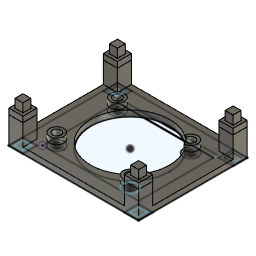
joyhv2 (Autodesk Fusion 360 design; units mm, degrees)
Autodesk Fusion 360 part; units mm, degrees
sketch "Sketch1" plane through (0, 0, 0) normal (0, 0, 1) x (1, 0, 0)
  line L0 (0, 0) -> (34, 0)
  line L1 (34, 0) -> (34, 26.5)
  line L2 (34, 26.5) -> (0, 26.5)
  line L3 (0, 26.5) -> (0, 0)
  line L4 (0, 26.5) -> (34, 26.5)
  line L5 (34, 26.5) -> (34, 28)
  line L6 (34, 28) -> (0, 28)
  line L7 (0, 28) -> (0, 26.5)
  circle A0 centre (28.5, 24) radius 1.5
  circle A1 centre (28.5, 2.5) radius 1.5
  circle A2 centre (2.5, 2.5) radius 1.5
  circle A3 centre (2.5, 24) radius 1.5
  circle A4 centre (16.5, 14.5) radius 14
  line L8 (-6, 32.5) -> (40, 32.5)
  line L9 (40, 32.5) -> (40, -6)
  line L10 (40, -6) -> (-6, -6)
  line L11 (-6, -6) -> (-6, 32.5)
  line L12 (40, 32.5) -> (35, 32.5)
  line L13 (35, 32.5) -> (35, 27.5)
  line L14 (35, 27.5) -> (40, 27.5)
  line L15 (40, 27.5) -> (40, 32.5)
  line L16 (40, -6) -> (35, -6)
  line L17 (35, -6) -> (35, -1)
  line L18 (35, -1) -> (40, -1)
  line L19 (40, -1) -> (40, -6)
  line L20 (-6, -6) -> (-1, -6)
  line L21 (-1, -6) -> (-1, -1)
  line L22 (-1, -1) -> (-6, -1)
  line L23 (-6, -1) -> (-6, -6)
  line L24 (-6, 32.5) -> (-1, 32.5)
  line L25 (-1, 32.5) -> (-1, 27.5)
  line L26 (-1, 27.5) -> (-6, 27.5)
  line L27 (-6, 27.5) -> (-6, 32.5)
  line L28 (-5, 31.5) -> (-2, 31.5)
  line L29 (-2, 31.5) -> (-2, 28.5)
  line L30 (-2, 28.5) -> (-5, 28.5)
  line L31 (-5, 28.5) -> (-5, 31.5)
  line L32 (-5, -2) -> (-2, -2)
  line L33 (-2, -2) -> (-2, -5)
  line L34 (-2, -5) -> (-5, -5)
  line L35 (-5, -5) -> (-5, -2)
  line L36 (36, -2) -> (39, -2)
  line L37 (39, -2) -> (39, -5)
  line L38 (39, -5) -> (36, -5)
  line L39 (36, -5) -> (36, -2)
  line L40 (36, 31.5) -> (39, 31.5)
  line L41 (39, 31.5) -> (39, 28.5)
  line L42 (39, 28.5) -> (36, 28.5)
  line L43 (36, 28.5) -> (36, 31.5)
  circle A5 centre (28.5, 2.5) radius 2.5
  circle A6 centre (28.5, 24) radius 2.5
  circle A7 centre (2.5, 2.5) radius 2.5
  circle A8 centre (2.5, 24) radius 2.5
  dimension "d1" = 34
  dimension "d2" = 26.5
  dimension "d3" = 1.5
  dimension "d4" = 3
  dimension "d5" = 3
  dimension "d6" = 3
  dimension "d7" = 3
  dimension "d8" = 2.5
  dimension "d9" = 2.5
  dimension "d10" = 2.5
  dimension "d11" = 5.5
  dimension "d12" = 5.5
  dimension "d13" = 2.5
  dimension "d14" = 2.5
  dimension "d15" = 2.5
  dimension "d16" = 28
  dimension "d17" = 16.5
  dimension "d18" = 6
  dimension "d19" = 6
  dimension "d20" = 6
  dimension "d21" = 6
  dimension "d22" = 5
  dimension "d23" = 5
  dimension "d24" = 5
  dimension "d25" = 5
  dimension "d26" = 5
  dimension "d27" = 5
  dimension "d28" = 5
  dimension "d29" = 5
  dimension "d30" = 1
  dimension "d31" = 1
  dimension "d32" = 3
  dimension "d33" = 1
  dimension "d34" = 1
  dimension "d35" = 5
  dimension "d36" = 5
  dimension "d37" = 5
  dimension "d77" = 14.5
  constraint horizontal L0
  constraint vertical L1
  constraint horizontal L2
  constraint vertical L3
  constraint coincident L0.start L3.end
  constraint horizontal L4
  constraint vertical L5
  constraint horizontal L6
  constraint vertical L7
  constraint horizontal L8
  constraint vertical L9
  constraint horizontal L10
  constraint vertical L11
  constraint horizontal L12
  constraint vertical L13
  constraint horizontal L14
  constraint vertical L15
  constraint horizontal L16
  constraint vertical L17
  constraint horizontal L18
  constraint vertical L19
  constraint horizontal L20
  constraint vertical L21
  constraint horizontal L22
  constraint vertical L23
  constraint horizontal L24
  constraint vertical L25
  constraint horizontal L26
  constraint vertical L27
  constraint horizontal L28
  constraint vertical L29
  constraint horizontal L30
  constraint vertical L31
  constraint horizontal L32
  constraint vertical L33
  constraint horizontal L34
  constraint vertical L35
  constraint horizontal L36
  constraint vertical L37
  constraint horizontal L38
  constraint vertical L39
  constraint horizontal L40
  constraint vertical L41
  constraint horizontal L42
  constraint vertical L43
  constraint concentric A1 A5
  constraint concentric A0 A6
  constraint concentric A2 A7
  constraint concentric A3 A8
  measures "d1" distance of L0.start L0.end
  measures "d2" distance of L0.start L2.end
  measures "d3" distance of L2.end L6.end
  measures "d4" diameter of A0
  measures "d5" diameter of A1
  measures "d6" diameter of A2
  measures "d7" diameter of A3
  measures "d8" distance of L2 A3.centre
  measures "d9" distance of L3 A3.centre
  measures "d10" distance of L2 A0.centre
  measures "d11" distance of L1 A0.centre
  measures "d12" distance of L1 A1.centre
  measures "d13" distance of L0 A1.centre
  measures "d14" distance of L0 A2.centre
  measures "d15" distance of L3 A2.centre
  measures "d16" diameter of A4
  measures "d17" distance of L3 A4.centre
  measures "d18" distance of L4 L8
  measures "d19" distance of L3 L11
  measures "d20" distance of L0 L10
  measures "d21" distance of L1 L9
  measures "d22" distance of L8.end L12.end
  measures "d23" distance of L8.end L14.end
  measures "d24" distance of L9.end L16.end
  measures "d25" distance of L9.end L18.end
  measures "d26" distance of L10.end L20.end
  measures "d27" distance of L10.end L22.end
  measures "d28" distance of L8.start L24.end
  measures "d29" distance of L8.start L26.end
  measures "d30" distance of L8 L28
  measures "d31" distance of L27 L31
  measures "d32" distance of L40.start L42.end
  measures "d33" distance of L8 L40
  measures "d34" distance of L13 L43
  measures "d35" diameter of A6
  measures "d36" diameter of A7
  measures "d37" diameter of A8
  measures "d77" distance of L0 A4.centre
extrude "Extrude1" add sketch "Sketch1" along normal blind 2 contours L0 L3 A7 | A5 | L0 L1 L2 L3 L4 A4 A6 A7 A8 | A7 | L2 L3 L4 A8 | A8 | L2 L4 L6 L7 A4 | L2 L4 L5 L6 A4 | L2 L4 A4 A6 | A0 A4 A6 | L8 L11 L24 L25 L26 L27 | L8 L9 L10 L11 L13 L14 L17 L18 L21 L22 L25 L26 | L8 L9 L12 L13 L14 L15 | L10 L11 L20 L21 L22 L23 | L9 L10 L16 L17 L18 L19 | L28 L29 L30 L31 | L32 L33 L34 L35 | L36 L37 L38 L39 | L40 L41 L42 L43 picked at (25.5001, 25.6456) picked at (26.5851, 24.6642) makes body 1
extrude "Extrude2" add sketch "Sketch1" along normal blind 4 contours A5 | A7 | A8 | A0 A4 A6 picked at (26.5851, 24.6642) bodies 1
extrude "Extrude3" add sketch "Sketch1" along normal blind 4 contours L8 L11 L24 L25 L26 L27 | L8 L9 L12 L13 L14 L15 | L10 L11 L20 L21 L22 L23 | L9 L10 L16 L17 L18 L19 | L28 L29 L30 L31 | L32 L33 L34 L35 | L36 L37 L38 L39 | L40 L41 L42 L43 bodies 1
extrude "Extrude4" add sketch "Sketch1" along normal blind 11.5 contours L8 L11 L24 L25 L26 L27 | L8 L9 L12 L13 L14 L15 | L10 L11 L20 L21 L22 L23 | L9 L10 L16 L17 L18 L19 bodies 1
move_body "Move1" bodies 1 to x (1, 0, 0) y (0, 1, 0) z (0, 0, 1) at (-61, 0, 0)
extrude "Extrude5" add sketch "Sketch1" along normal blind 2 separate body contours L0 L3 A7 | A5 | L0 L1 L2 L3 L4 A4 A6 A7 A8 | A7 | L2 L3 L4 A8 | A8 | L2 L4 L6 L7 A4 | L2 L4 L5 L6 A4 | L2 L4 A4 A6 | A0 A4 A6 | A0 A4 | A1 | A2 | A3 | L8 L11 L24 L25 L26 L27 | L8 L9 L10 L11 L13 L14 L17 L18 L21 L22 L25 L26 | L8 L9 L12 L13 L14 L15 | L10 L11 L20 L21 L22 L23 | L9 L10 L16 L17 L18 L19 | L28 L29 L30 L31 | L32 L33 L34 L35 | L36 L37 L38 L39 | L40 L41 L42 L43 picked at (25.5001, 25.6456) picked at (26.5851, 24.6642) picked at (28.192, 23.7895) makes body 2
extrude "Extrude6" add sketch "Sketch1" along normal blind 9.5 contours L8 L11 L24 L25 L26 L27 | L8 L9 L12 L13 L14 L15 | L10 L11 L20 L21 L22 L23 | L9 L10 L16 L17 L18 L19 | L28 L29 L30 L31 | L32 L33 L34 L35 | L36 L37 L38 L39 | L40 L41 L42 L43 bodies 2
sketch "Sketch2" plane through (0, 0, 9.5) normal (0, 0, 1) x (-1, 0, 0)
  line L0 (6, -27.5) -> (1, -27.5)
  line L1 (1, -27.5) -> (1, -32.5)
  line L2 (1, -32.5) -> (6, -32.5)
  line L3 (6, -32.5) -> (6, -27.5)
  line L4 (4.9, -31.4) -> (2.1, -31.4)
  line L5 (2.1, -31.4) -> (2.1, -28.6)
  line L6 (2.1, -28.6) -> (4.9, -28.6)
  line L7 (4.9, -28.6) -> (4.9, -31.4)
  line L8 (6, -27.5) -> (6, -32.5)
  line L9 (6, -32.5) -> (-40, -32.5)
  dimension "d50" = 2.8
  dimension "d51" = 2.8
  dimension "d52" = 1.1
  dimension "d53" = 1.1
  constraint horizontal L4
  constraint vertical L5
  constraint horizontal L6
  constraint vertical L7
  measures "d50" distance of L4.start L4.end
  measures "d51" distance of L4.start L6.end
  measures "d52" distance of L7 L8
  measures "d53" distance of L4 L9
sketch "Sketch3" plane through (0, 0, 9.5) normal (0, 0, 1) x (-1, 0, 0)
  line L0 (-40, -27.5) -> (-40, -32.5)
  line L1 (-40, -32.5) -> (-35, -32.5)
  line L2 (-35, -32.5) -> (-35, -27.5)
  line L3 (-35, -27.5) -> (-40, -27.5)
  line L4 (-36.1, -31.4) -> (-38.9, -31.4)
  line L5 (-38.9, -31.4) -> (-38.9, -28.6)
  line L6 (-38.9, -28.6) -> (-36.1, -28.6)
  line L7 (-36.1, -28.6) -> (-36.1, -31.4)
  line L8 (6, -32.5) -> (-40, -32.5)
  line L9 (-40, -27.5) -> (-40, -32.5)
  dimension "d54" = 2.8
  dimension "d55" = 2.8
  dimension "d56" = 1.1
  dimension "d57" = 1.1
  constraint horizontal L4
  constraint vertical L5
  constraint horizontal L6
  constraint vertical L7
  measures "d54" distance of L4.start L4.end
  measures "d55" distance of L4.start L6.end
  measures "d56" distance of L4 L8
  measures "d57" distance of L5 L9
sketch "Sketch4" plane through (0, 0, 9.5) normal (0, 0, 1) x (-1, 0, 0)
  line L0 (-40, 1) -> (-35, 1)
  line L1 (-35, 1) -> (-35, 6)
  line L2 (-35, 6) -> (-40, 6)
  line L3 (-40, 6) -> (-40, 1)
  line L4 (-36.1, 2.1) -> (-38.9, 2.1)
  line L5 (-38.9, 2.1) -> (-38.9, 4.9)
  line L6 (-38.9, 4.9) -> (-36.1, 4.9)
  line L7 (-36.1, 4.9) -> (-36.1, 2.1)
  line L8 (-35, 1) -> (-40, 1)
  line L9 (-40, -32.5) -> (-40, 6)
  dimension "d58" = 2.8
  dimension "d59" = 2.8
  dimension "d60" = 1.1
  dimension "d61" = 1.1
  constraint horizontal L4
  constraint vertical L5
  constraint horizontal L6
  constraint vertical L7
  measures "d58" distance of L4.start L4.end
  measures "d59" distance of L4.start L6.end
  measures "d60" distance of L4 L8
  measures "d61" distance of L5 L9
sketch "Sketch5" plane through (0, 0, 9.5) normal (0, 0, 1) x (-1, 0, 0)
  line L0 (6, 1) -> (6, 6)
  line L1 (6, 6) -> (1, 6)
  line L2 (1, 6) -> (1, 1)
  line L3 (1, 1) -> (6, 1)
  line L4 (4.9, 2.1) -> (2.1, 2.1)
  line L5 (2.1, 2.1) -> (2.1, 4.9)
  line L6 (2.1, 4.9) -> (4.9, 4.9)
  line L7 (4.9, 4.9) -> (4.9, 2.1)
  line L8 (1, 1) -> (6, 1)
  line L9 (6, 6) -> (6, -32.5)
  dimension "d62" = 2.8
  dimension "d63" = 2.8
  dimension "d64" = 1.1
  dimension "d65" = 1.1
  constraint horizontal L4
  constraint vertical L5
  constraint horizontal L6
  constraint vertical L7
  measures "d62" distance of L4.start L4.end
  measures "d63" distance of L4.start L6.end
  measures "d64" distance of L4 L8
  measures "d65" distance of L7 L9
extrude "Extrude7" add sketch "Sketch2" sketch "Sketch3" sketch "Sketch4" sketch "Sketch5" along normal blind 5 contours L4 L5 L6 L7 of sketch 2 contours L4 L5 L6 L7 of sketch 3 contours L4 L5 L6 L7 of sketch 4 contours L4 L5 L6 L7 bodies 2
sketch "Sketch6" plane through (0, 0, 2) normal (0, 0, 1) x (-1, 0, 0)
  circle A0 centre (-16.5, -14.5) radius 14
  line L0 (-35, 6) -> (-35, 1)
  line L1 (-35, 1) -> (-40, 1)
  line L2 (-40, 1) -> (-40, -27.5)
  line L3 (-40, -27.5) -> (-35, -27.5)
  line L4 (-35, -27.5) -> (-35, -32.5)
  line L5 (-35, -32.5) -> (1, -32.5)
  line L6 (1, -32.5) -> (1, -27.5)
  line L7 (1, -27.5) -> (6, -27.5)
  line L8 (6, -27.5) -> (6, 1)
  line L9 (6, 1) -> (1, 1)
  line L10 (1, 1) -> (1, 6)
  line L11 (1, 6) -> (-35, 6)
  circle A1 centre (-16.5, -14.5) radius 14
  line L12 (-16.5, -28.5) -> (-16.5, -0.5)
  circle A2 centre (-16.5, -14.5) radius 15
  line L13 (-16.5, -29.5) -> (-16.5, 0.5)
  dimension "d68" = 30
  constraint concentric A0 A1
  constraint coincident A1 L12.start
  constraint coincident A1 L12.end
  constraint vertical L12
  constraint concentric A1 A2
  constraint coincident A2 L13.start
  constraint coincident A2 L13.end
  constraint parallel L12 L13
  measures "d68" diameter of A2
revolve "Revolve1" add sketch "Sketch6" angle 180 about axis through (16.5, 28.5, 2) along (0, 1, 0) contours A0 A1 A2 L13 picked at (-17.2452, 0.1108) bodies 2
sketch "Sketch7" plane through (0, -6, 0) normal (0, -1, 0) x (1, 0, 0)
  line L0 (35, 2) -> (-1, 2)
  line L1 (-1, 2) -> (-1, 9.5)
  line L2 (-1, 9.5) -> (-6, 9.5)
  line L3 (-6, 9.5) -> (-6, 0)
  line L4 (-6, 0) -> (40, 0)
  line L5 (40, 0) -> (40, 9.5)
  line L6 (40, 9.5) -> (35, 9.5)
  line L7 (35, 9.5) -> (35, 2)
  line L8 (0, 0) -> (34, 0)
  line L9 (34, 0) -> (34, -3)
  line L10 (34, -3) -> (0, -3)
  line L11 (0, -3) -> (0, 0)
  line L12 (0, -3) -> (34, -3)
  line L13 (34, -3) -> (34, -14)
  line L14 (34, -14) -> (0, -14)
  line L15 (0, -14) -> (0, -3)
  dimension "d70" = 3
  constraint horizontal L8
  constraint vertical L9
  constraint horizontal L10
  constraint vertical L11
  constraint coincident L8.start L11.end
  constraint horizontal L12
  constraint vertical L13
  constraint horizontal L14
  constraint vertical L15
  measures "d70" distance of L8.start L10.end
extrude "Extrude8" cut sketch "Sketch7" against normal blind 44 contours L10 L12 L13 L14 L15 bodies 2
fillet "Fillet1" radius 1.5 1 edges at (21.614, 1.3149, -3) on bodies 2
sketch "Sketch8" plane through (0, 32.5, 0) normal (0, 1, 0) x (-1, 0, 0)
  line L0 (-40, 0) -> (6, 0)
  line L1 (6, 0) -> (6, 9.5)
  line L2 (6, 9.5) -> (1, 9.5)
  line L3 (1, 9.5) -> (1, 2)
  line L4 (1, 2) -> (-35, 2)
  line L5 (-35, 2) -> (-35, 9.5)
  line L6 (-35, 9.5) -> (-40, 9.5)
  line L7 (-40, 9.5) -> (-40, 0)
  line L8 (-32.6127, 0) -> (-1, 0)
  line L9 (-1, 0) -> (-1, -6)
  line L10 (-1, -6) -> (-32.6127, -6)
  line L11 (-32.6127, -6) -> (-32.6127, 0)
  constraint horizontal L8
  constraint vertical L9
  constraint horizontal L10
  constraint vertical L11
  constraint coincident L0 L8.start
extrude "Extrude9" cut sketch "Sketch8" against normal blind 47 contours L0 L8 L9 L10 L11 bodies 2
move_body "Move2" bodies 1 to x (1, 0, 0) y (0, 1, 0) z (0, 0, 1) at (61, 0, 0)
equation "d44 = 4 mm + 7.5 mm"
